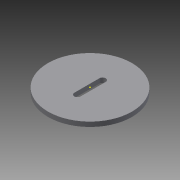
# Autodesk Inventor part: midCup
Saved by Autodesk Inventor 2015 (Build 190159000, 159)
## iProperties
Created: 2015-02-13
Part Number: midCup
Material: Generic
Document SubType Name: Modeling
Designer: Qiuyang
Density: 1 g/cm^3
Appearance: Default
Author: Qiuyang
Autodesk Inventor part; units mm, degrees
ref_plane "YZ Plane" through (0, 0, 0) normal (1, 0, 0) x (0, 1, 0)
ref_plane "XZ Plane" through (0, 0, 0) normal (0, 1, 0) x (-1, 0, 0)
ref_plane "XY Plane" through (0, 0, 0) normal (0, 0, 1) x (1, 0, 0)
sketch "Sketch1" plane through (0, 0, 0) normal (0, 1, 0) x (-1, 0, 0)
  circle A0 centre (0, 0) radius 50.8
  dimension "d0" = 101.6
  constraints: 1 centre point, 1 coincident
  measures "d0" diameter of A0
extrude "Extrusion1" add sketch "Sketch1" along normal blind 5.588
sketch "Sketch2" plane through (0, 5.588, 0) normal (0, 1, 0) x (1, 0, 0)
  line L0 (3.81, 13.97) -> (-3.81, 13.97)
  line L1 (-3.81, 13.97) -> (-3.81, -13.97)
  line L2 (-3.81, -13.97) -> (3.81, -13.97)
  line L3 (3.81, -13.97) -> (3.81, 13.97)
  point P0 (0, 0)
  dimension "d3" = 7.62
  dimension "d4" = 27.94
  constraints: 8 end point, 2 parallel, 1 horizontal, 1 perpendicular
  measures "d3" distance of L2.end L1.end
  measures "d4" distance of L1.end L0.end
extrude "Extrusion2" cut sketch "Sketch2" against normal blind 5.588
sketch "Sketch3" plane through (0, 5.588, 0) normal (0, 1, 0) x (1, 0, 0)
  point P0 (0, 0)
sketch "Sketch4" plane through (0, 5.588, 0) normal (0, 1, 0) x (1, 0, 0)
  line L0 (3.81, 15.24) -> (-3.81, 15.24)
  line L1 (-3.81, 15.24) -> (-3.81, -15.24)
  line L2 (-3.81, -15.24) -> (3.81, -15.24)
  line L3 (3.81, -15.24) -> (3.81, 15.24)
  point P0 (0, 0)
  dimension "d7" = 30.48
  constraints: 8 end point, 2 parallel, 1 horizontal, 1 perpendicular
  measures "d7" distance of L1.end L0.end
extrude "Extrusion3" cut sketch "Sketch4" against normal blind 5.588
sketch "Sketch5" plane through (0, 5.588, 0) normal (0, 1, 0) x (1, 0, 0)
  line L0 (3.81, 15.24) -> (-3.81, 15.24) projected
  circle A0 centre (0, 15.24) radius 3.81
  point P0 (0, 0)
  dimension "d10" = 7.62
  constraints: 1 centre point, 1 midpoint
  measures "d10" diameter of A0
extrude "Extrusion4" cut sketch "Sketch5" against normal blind 5.588
sketch "Sketch6" plane through (0, 5.588, 0) normal (0, 1, 0) x (1, 0, 0)
  line L0 (-3.81, -15.24) -> (3.81, -15.24) projected
  circle A0 centre (0, -15.24) radius 3.81
  point P0 (0, 0)
  dimension "d13" = 7.62
  constraints: 1 centre point, 1 midpoint
  measures "d13" diameter of A0
extrude "Extrusion5" cut sketch "Sketch6" against normal blind 5.588
sketch "Sketch7" plane through (0, 5.588, 0) normal (0, 1, 0) x (1, 0, 0)
  point P0 (0, 0)
body "Solid1"
